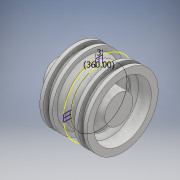
# Autodesk Inventor part: Wheel Rim
Saved by Autodesk Inventor 2018 (Build 220112000, 112)
## iProperties
Created: 2019-07-12
Part Number: Wheel Rim
Material: Generic
Document SubType Name: Modeling
Designer: Ngo Sin Siong
Density: 1 g/cm^3
Appearance: Default
Author: Ngo Sin Siong
Autodesk Inventor part; units mm, degrees
ref_plane "YZ Plane" through (0, 0, 0) normal (1, 0, 0) x (0, 1, 0)
ref_plane "XZ Plane" through (0, 0, 0) normal (0, 1, 0) x (-1, 0, 0)
ref_plane "XY Plane" through (0, 0, 0) normal (0, 0, 1) x (1, 0, 0)
sketch "Sketch1" plane through (0, 0, 0) normal (0, 1, 0) x (-1, 0, 0)
  line L0 (0, 0) -> (10.1, 0) construction
  line L1 (10.1, 0) -> (10.1, -10.9) construction
  line L2 (10.1, -10.9) -> (0, -10.9) construction
  line L3 (0, -10.9) -> (0, 0) construction
  line L4 (10.1, 0) -> (4.6, 0) construction
  line L5 (4.6, 0) -> (4.6, -12.3) construction
  line L6 (4.6, -12.3) -> (10.1, -12.3) construction
  line L7 (10.1, -12.3) -> (10.1, 0) construction
  line L8 (4.6, -10.9) -> (2.6, -10.9) construction
  line L9 (2.6, -10.9) -> (4.6, -12.3) construction
  line L10 (0, 0) -> (17.75, 0) construction
  line L11 (17.75, 0) -> (17.75, -6) construction
  line L12 (17.75, -6) -> (0, -6) construction
  line L13 (0, -6) -> (0, 0) construction
  line L14 (10.1, 0) -> (8.5, 0) construction
  line L15 (8.5, 0) -> (8.5, -15.2) construction
  line L16 (8.5, -15.2) -> (10.1, -15.2) construction
  line L17 (10.1, -15.2) -> (10.1, 0) construction
  line L18 (8.5, 0) -> (6.2, 0) construction
  line L19 (6.2, 0) -> (6.2, -13.2) construction
  line L20 (6.2, -13.2) -> (8.5, -13.2) construction
  line L21 (8.5, -13.2) -> (8.5, 0) construction
  line L22 (0, 0) -> (0, -12) construction
  line L23 (0, -12) -> (2.6, -12) construction
  line L24 (6.2, 0) -> (4.6, 0) construction
  line L25 (4.6, 0) -> (4.6, -15.2) construction
  line L26 (4.6, -15.2) -> (6.2, -15.2) construction
  line L27 (6.2, -15.2) -> (6.2, 0) construction
  line L28 (4.6, -15.2) -> (4.6, -13.3) construction
  line L29 (4.6, -13.3) -> (2.6, -12) construction
  line L30 (0, 0) -> (-10.1, 0) construction
  line L31 (-10.1, 0) -> (-10.1, -10.9) construction
  line L32 (-10.1, -10.9) -> (0, -10.9) construction
  line L33 (-10.1, 0) -> (-4.6, 0) construction
  line L34 (-4.6, 0) -> (-4.6, -12.3) construction
  line L35 (-4.6, -12.3) -> (-10.1, -12.3) construction
  line L36 (-10.1, -12.3) -> (-10.1, 0) construction
  line L37 (-4.6, -10.9) -> (-2.6, -10.9) construction
  line L38 (-2.6, -10.9) -> (-4.6, -12.3) construction
  line L39 (-10.1, 0) -> (-8.5, 0) construction
  line L40 (-8.5, 0) -> (-8.5, -15.2) construction
  line L41 (-8.5, -15.2) -> (-10.1, -15.2) construction
  line L42 (-10.1, -15.2) -> (-10.1, 0) construction
  line L43 (-8.5, 0) -> (-6.2, 0) construction
  line L44 (-6.2, 0) -> (-6.2, -13.2) construction
  line L45 (-6.2, -13.2) -> (-8.5, -13.2) construction
  line L46 (-8.5, -13.2) -> (-8.5, 0) construction
  line L47 (0, -12) -> (-2.6, -12) construction
  line L48 (-6.2, 0) -> (-4.6, 0) construction
  line L49 (-4.6, 0) -> (-4.6, -15.2) construction
  line L50 (-4.6, -15.2) -> (-6.2, -15.2) construction
  line L51 (-6.2, -15.2) -> (-6.2, 0) construction
  line L52 (-4.6, -15.2) -> (-4.6, -13.3) construction
  line L53 (-4.6, -13.3) -> (-2.6, -12) construction
  line L54 (0, 0) -> (-2, 0) construction
  line L55 (-2, 0) -> (-2, -10.9) construction
  line L56 (-2, -10.9) -> (0, -10.9) construction
  line L57 (0, -10.9) -> (0, 0) construction
  line L58 (0, 0) -> (2, 0) construction
  line L59 (2, 0) -> (2, -10.9) construction
  line L60 (2, -10.9) -> (0, -10.9) construction
  line L61 (0, -10.9) -> (0, 0) construction
  line L62 (0, -6) -> (-8.5, -6) construction
  line L63 (-8.5, -6) -> (-8.5, 0) construction
  line L64 (-8.5, 0) -> (0, 0) construction
  line L65 (0, 0) -> (0, -6) construction
  line L66 (10.1, -12.3) -> (8.5, -12.3) construction
  line L67 (8.5, -12.3) -> (6.2, -12.3) construction
  line L68 (4.6, -12.3) -> (4.6, -13.3) construction
  line L69 (2.6, -12) -> (2.6, -10.9) construction
  line L70 (-2.6, -10.9) -> (-4.6, -12.3) construction
  line L71 (-6.2, -12.3) -> (-8.5, -12.3) construction
  line L72 (-10.1, -12.3) -> (-10.1, -15.2) construction
  line L73 (-8.5, -15.2) -> (-8.5, -13.2) construction
  line L74 (-6.2, -13.2) -> (-6.2, -15.2) construction
  line L75 (10.1, -12.3) -> (4.6, -12.3) construction
  line L76 (2.6, -10.9) -> (2, -10.9) construction
  line L77 (2, -6) -> (17.75, -6) construction
  line L78 (17.75, 0) -> (-8.5, 0) construction
  line L79 (-8.5, -6) -> (-2, -6) construction
  line L80 (-2, -10.9) -> (-2.6, -10.9) construction
  line L81 (-4.6, -12.3) -> (-10.1, -12.3) construction
  line L82 (-10.1, -15.2) -> (-8.5, -15.2) construction
  line L83 (17.75, 0) -> (17.75, -6)
  line L84 (2, -6) -> (2, -10.9)
  line L85 (2.6, -10.9) -> (4.6, -12.3)
  line L86 (10.1, -12.3) -> (10.1, -15.2)
  line L87 (8.5, -15.2) -> (8.5, -13.2)
  line L88 (6.2, -13.2) -> (6.2, -15.2)
  line L89 (4.6, -15.2) -> (4.6, -13.3)
  line L90 (2.6, -12) -> (-2.6, -12)
  line L91 (-4.6, -13.3) -> (-4.6, -15.2)
  line L92 (-6.2, -15.2) -> (-6.2, -13.2)
  line L93 (-8.5, -13.2) -> (-8.5, -15.2)
  line L94 (-10.1, -15.2) -> (-10.1, -12.3)
  line L95 (-6.2, -13.2) -> (-8.5, -13.2)
  line L96 (-2.6, -12) -> (-4.6, -13.3)
  line L97 (-4.6, -12.3) -> (-10.1, -12.3)
  line L98 (4.6, -13.3) -> (2.6, -12)
  line L99 (4.6, -15.2) -> (6.2, -15.2)
  line L100 (-4.6, -12.3) -> (-2.6, -10.9)
  line L101 (-2, -10.9) -> (-2.6, -10.9)
  line L102 (-2, -6) -> (-2, -10.9)
  line L103 (8.5, -13.2) -> (6.2, -13.2)
  line L104 (8.5, -15.2) -> (10.1, -15.2)
  line L105 (10.1, -12.3) -> (4.6, -12.3)
  line L106 (17.75, -6) -> (2, -6)
  line L107 (17.75, 0) -> (-8.5, 0)
  line L108 (-8.5, -6) -> (-8.5, 0)
  line L109 (-8.5, -6) -> (-2, -6)
  line L110 (-4.6, -15.2) -> (-6.2, -15.2)
  line L111 (-8.5, -15.2) -> (-10.1, -15.2)
  line L112 (-2, -6) -> (-8.5, -6)
  line L113 (-8.5, -6) -> (-8.5, -7)
  line L114 (-8.5, -7) -> (-2, -7)
  line L115 (-2, -7) -> (-2, -6)
  line L116 (2, -6) -> (17.75, -6)
  line L117 (17.75, -6) -> (17.75, -7)
  line L118 (17.75, -7) -> (2, -7)
  line L119 (2, -7) -> (2, -6)
  line L120 (2.6, -10.9) -> (2, -10.9)
  dimension "d0" = 10.1
  dimension "d1" = 10.9
  dimension "d2" = 5.5
  dimension "d3" = 12.3
  dimension "d4" = 2
  dimension "d5" = 17.75
  dimension "d6" = 6
  dimension "d7" = 1.6
  dimension "d8" = 15.2
  dimension "d9" = 2.3
  dimension "d10" = 13.2
  dimension "d12" = 12
  dimension "d13" = 2.6
  dimension "d15" = 15.2
  dimension "d16" = 1.9
  dimension "d17" = 2
  dimension "d18" = 2
  dimension "d19" = 1
  dimension "d20" = 1
  constraints: 242 end point, 31 parallel, 24 collinear, 24 point on line, 18 perpendicular, 17 symmetric about line, 13 horizontal
  measures "d0" distance of L1.end L2.end
  measures "d1" distance of L0.end L1.end
  measures "d2" distance of L6.end L5.end
  measures "d3" distance of L4.end L5.end
  measures "d4" distance of L8.start L8.end
  measures "d5" distance of L11.end L12.end
  measures "d6" distance of L10.end L11.end
  measures "d7" distance of L16.end L15.end
  measures "d8" distance of L15.end L14.end
  measures "d9" distance of L20.end L19.end
  measures "d10" distance of L19.end L18.end
  measures "d12" distance of L0.start L22.end
  measures "d13" distance of L22.end L23.end
  measures "d15" distance of L25.end L4.end
  measures "d16" distance of L25.end L28.end
  measures "d17" distance of L56.end L55.end
  measures "d18" distance of L59.end L60.end
  measures "d19" distance of L113.end L112.end
  measures "d20" distance of L116.end L117.end
revolve "Revolution1" add sketch "Sketch1" angle 360 about axis through (0, 0, 0) along (-1, 0, 0) contours L83 L106 L84 L120 L85 L105 L86 L104 L87 L103 L88 L99 L89 L98 L90 L96 L91 L110 L92 L95 L93 L111 L94 L97 L100 L101 L102 L109 L108 L107
sketch "Sketch2" plane through (0, 0, 0) normal (1, 0, 0) x (0, 1, 0)
  line L0 (0, 0) -> (0, 12)
  circle A0 centre (0, 0) radius 12 projected
  line L1 (0, 12) -> (0, 15.2)
  circle A1 centre (0, 0) radius 15.2 projected
  line L2 (-1.5, 15.2) -> (1.5, 15.2)
  line L3 (-1.5, 15.2) -> (0, 15.2)
  line L4 (0, 15.2) -> (0, 0)
  line L5 (0, 0) -> (-1.5, 0)
  line L6 (-1.5, 0) -> (-1.5, 15.2)
  line L7 (0, 0) -> (1.5, 0)
  line L8 (1.5, 0) -> (1.5, 15.2)
  line L9 (1.5, 15.2) -> (0, 15.2)
  line L10 (0, 15.2) -> (0, 0)
  line L11 (0, 0) -> (-12, 0)
  line L12 (-12, 0) -> (-15.2, 0)
  line L13 (-15.2, -1.5) -> (-15.2, 1.5)
  line L14 (-15.2, -1.5) -> (-15.2, 0)
  line L15 (-15.2, 0) -> (0, 0)
  line L16 (0, 0) -> (0, -1.5)
  line L17 (0, -1.5) -> (-15.2, -1.5)
  line L18 (0, 0) -> (0, 1.5)
  line L19 (0, 1.5) -> (-15.2, 1.5)
  line L20 (-15.2, 1.5) -> (-15.2, 0)
  line L21 (-15.2, 0) -> (0, 0)
  line L22 (0, 0) -> (0, -12)
  line L23 (0, -12) -> (0, -15.2)
  line L24 (1.5, -15.2) -> (-1.5, -15.2)
  line L25 (1.5, -15.2) -> (0, -15.2)
  line L26 (0, -15.2) -> (0, 0)
  line L27 (0, 0) -> (1.5, 0)
  line L28 (1.5, 0) -> (1.5, -15.2)
  line L29 (0, 0) -> (-1.5, 0)
  line L30 (-1.5, 0) -> (-1.5, -15.2)
  line L31 (-1.5, -15.2) -> (0, -15.2)
  line L32 (0, -15.2) -> (0, 0)
  line L33 (0, 0) -> (12, 0)
  line L34 (12, 0) -> (15.2, 0)
  line L35 (15.2, 1.5) -> (15.2, -1.5)
  line L36 (15.2, 1.5) -> (15.2, 0)
  line L37 (15.2, 0) -> (0, 0)
  line L38 (0, 0) -> (0, 1.5)
  line L39 (0, 1.5) -> (15.2, 1.5)
  line L40 (0, 0) -> (0, -1.5)
  line L41 (0, -1.5) -> (15.2, -1.5)
  line L42 (15.2, -1.5) -> (15.2, 0)
  line L43 (15.2, 0) -> (0, 0)
  dimension "d22" = 3
  dimension "d25" = 360
  constraints: 88 end point, 4 parallel, 3 horizontal, 2 coincident, 2 perpendicular, 2 vertical, 2 vertical alignment, 1 midpoint, 89 other
  measures "d22" distance of L2.start L2.end
body "Solid1"
